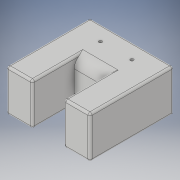
# Autodesk Inventor part: stand_holder
Saved by Autodesk Inventor 2019 (Build 230136000, 136)
## iProperties
Created: 2019-12-27
Part Number: stand_holder
Material: Типовые
Document SubType Name: Modeling
Designer: stepa
Density: 1 g/cm^3
Appearance: По умолчанию
Author: stepa
Autodesk Inventor part; units mm, degrees
ref_plane "YZ Plane" through (0, 0, 0) normal (1, 0, 0) x (0, 1, 0)
ref_plane "XZ Plane" through (0, 0, 0) normal (0, 1, 0) x (-1, 0, 0)
ref_plane "XY Plane" through (0, 0, 0) normal (0, 0, 1) x (1, 0, 0)
sketch "Эскиз1" plane through (0, 0, 0) normal (0, 1, 0) x (-1, 0, 0)
  line L0 (29.5774, -51.5004) -> (-50.4226, -51.5004)
  line L1 (-50.4226, -51.5004) -> (-50.4226, 28.4996)
  line L2 (-50.4226, 28.4996) -> (-25.4226, 28.4996)
  line L3 (-25.4226, 28.4996) -> (-25.4226, -11.5004)
  line L4 (-25.4226, -11.5004) -> (4.5774, -11.5004)
  line L5 (4.5774, -11.5004) -> (4.5774, 28.4996)
  line L6 (4.5774, 28.4996) -> (29.5774, 28.4996)
  line L7 (29.5774, 28.4996) -> (29.5774, -51.5004)
  point P0 (0, 0)
  dimension "d0" = 30
  dimension "d1" = 80
  dimension "d2" = 40
  dimension "d3" = 80
  constraints: 16 end point, 6 perpendicular, 2 point on line, 1 collinear, 1 horizontal
  measures "d0" distance of L3.end L4.end
  measures "d1" distance of L0.start L0.end
  measures "d2" distance between parallel lines of L0 L4
  measures "d3" distance of L6.end L0.start
extrude "Выдавливание1" add sketch "Эскиз1" along normal blind 40
fillet "Сопряжение1" radius 10 2 edges at (10.4226, 40, -11.5004) (10.4226, 0, -11.5004)
fillet "Сопряжение2" radius 2 19 edges at (10.4226, 40, -51.5004) (-29.5774, 20, -51.5004) (50.4226, 20, -51.5004) (-17.0774, 40, 28.4996) (37.9226, 40, 28.4996) (37.9226, 0, 28.4996) (-17.0774, 0, 28.4996) (-4.5774, 40, 8.4996) (-29.5774, 40, -11.5004) (-29.5774, 0, -11.5004) (-29.5774, 20, 28.4996) (-4.5774, 20, 28.4996) (25.4226, 40, 8.4996) (25.4226, 20, 28.4996) (25.4226, 0, 8.4996) (-4.5774, 0, 8.4996) (50.4226, 20, 28.4996) (50.4226, 0, -11.5004) (50.4226, 40, -11.5004)
sketch "Эскиз2" plane through (0, 0, 0) normal (0, -1, 0) x (1, 0, 0)
  line L0 (-29.5774, 26.4996) -> (-29.5774, -49.5004) projected
  line L1 (-27.5774, -51.5004) -> (48.4226, -51.5004) projected
  point P0 (0, 0)
  point P1 (-4.5774, -36.5004)
  point P2 (25.4226, -36.5004)
  dimension "d8" = 30
  dimension "d9" = 25
  dimension "d10" = 15
  constraints: 1 horizontal alignment
  measures "d8" distance of point (25.423, -36.5) point (-4.577, -36.5)
  measures "d9" distance from line of L0 point (-4.577, -36.5)
  measures "d10" distance from line of L1 point (-4.577, -36.5)
hole "Отверстие1" at (-4.5774, 0, -36.5004) at (25.4226, 0, -36.5004) direction (0, 1, 0) diameter 3 end through all
